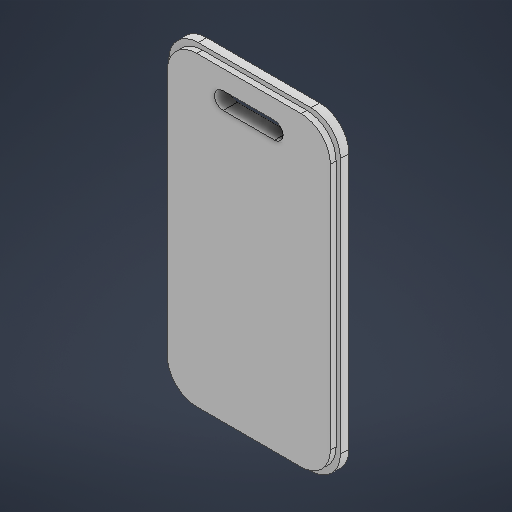
# Autodesk Inventor part: BackPlate
Saved by Autodesk Inventor 2026 (Build 300175050, 175E)
## iProperties
Created: 2026-03-28
Part Number: BackPlate
Material: Generic
Document SubType Name: Modeling
Designer: tp2105
Density: 1 g/cm^3
Appearance: Default
Author: tp2105
Autodesk Inventor part; units mm, degrees
ref_plane "YZ Plane" through (0, 0, 0) normal (1, 0, 0) x (0, 1, 0)
ref_plane "XZ Plane" through (0, 0, 0) normal (0, 1, 0) x (-1, 0, 0)
ref_plane "XY Plane" through (0, 0, 0) normal (0, 0, 1) x (1, 0, 0)
sketch "Sketch1" plane through (0, 0, 0) normal (0, 0, 1) x (1, 0, 0)
  line L0 (0, 0) -> (64.8574, 0) construction
  line L1 (-30, -55) -> (30, -55)
  line L2 (30, -55) -> (30, 55)
  line L3 (30, 55) -> (-30, 55)
  line L4 (-30, 55) -> (-30, -55)
  line L5 (-30, -55) -> (30, 55) construction
  line L6 (30, -55) -> (-30, 55) construction
  dimension "d0" = 60
  dimension "d1" = 110
  constraints: 14 end point, 2 horizontal, 2 midpoint, 2 parallel, 1 coincident, 1 perpendicular
  measures "d0" distance of L3.end L2.end
  measures "d1" distance of L2.end L1.end
extrude "Extrusion1" add sketch "Sketch1" along normal blind 3
fillet "Fillet1" radius 10.25 4 edges at (30, 55, 1.5) (-30, 55, 1.5) (30, -55, 1.5) (-30, -55, 1.5)
sketch "Sketch2" plane through (0, 0, 3) normal (0, 0, 1) x (1, 0, 0)
  line L0 (0, 0) -> (47.0336, 0) construction
  line L1 (-30, -55) -> (30, -55)
  line L2 (30, -55) -> (30, 55)
  line L3 (30, 55) -> (-30, 55)
  line L4 (-30, 55) -> (-30, -55)
  line L5 (-30, -55) -> (30, 55) construction
  line L6 (30, -55) -> (-30, 55) construction
  line L7 (-28.5, 53.5) -> (28.5, 53.5)
  line L8 (28.5, 53.5) -> (28.5, -53.5)
  line L9 (28.5, -53.5) -> (-28.5, -53.5)
  line L10 (-28.5, -53.5) -> (-28.5, 53.5)
  dimension "d5" = 60
  dimension "d6" = 110
  dimension "d7" = 1.5
  constraints: 22 end point, 4 parallel, 2 coincident, 2 horizontal, 2 midpoint, 2 perpendicular, 3 other
  measures "d5" distance of L3.end L2.end
  measures "d6" distance of L2.end L1.end
  measures "d7" distance between parallel lines of L3 L7
extrude "Extrusion2" add sketch "Sketch2" along normal blind 2 contours L7 L8 L9 L10
fillet "Fillet2" radius 10.25 4 edges at (28.5, 53.5, 4) (-28.5, 53.5, 4) (-28.5, -53.5, 4) (28.5, -53.5, 4)
sketch "Sketch3" plane through (0, 0, 0) normal (0, 0, -1) x (-1, 0, 0)
  line L0 (9, 43.8265) -> (-9, 43.8265) construction
  line L1 (9, 45.3265) -> (-9, 45.3265)
  line L2 (-9, 42.3265) -> (9, 42.3265)
  arc A0 (9, 42.3265) -> (9, 45.3265) centre (9, 43.8265) ccw
  arc A1 (-9, 45.3265) -> (-9, 42.3265) centre (-9, 43.8265) ccw
  line L3 (-9, 46.8265) -> (9, 46.8265)
  arc A2 (9, 40.8265) -> (9, 46.8265) centre (9, 43.8265) ccw
  line L4 (9, 40.8265) -> (-9, 40.8265)
  arc A3 (-9, 46.8265) -> (-9, 40.8265) centre (-9, 43.8265) ccw
  point P0 (0, 0)
  point P1 (0, 43.8265)
  dimension "d11" = 9
  dimension "d12" = 3
  dimension "d15" = 1.5
  constraints: 12 end point, 8 point on circle, 4 centre point, 4 tangent, 2 parallel, 1 horizontal, 1 midpoint, 3 other
  measures "d11" distance of point (0, 43.826) L0.end
  measures "d12" diameter of A1
  measures "d15" distance between parallel lines of L1 L3
extrude "Extrusion3" cut sketch "Sketch3" against normal through all contours A0 L2 A1 L1 | L3 A2 L4 A3
sketch "Sketch4" plane through (0, 0, 4) normal (0, 0, -1) x (-1, 0, 0)
  point P0 (0, 0)
body "Solid1"
